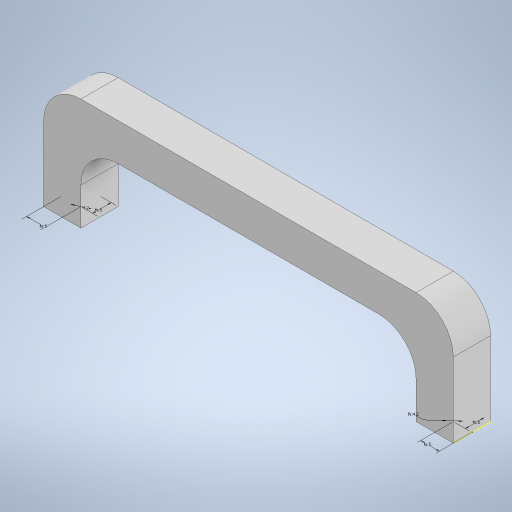
# Autodesk Inventor part: side door handle v02
Saved by Autodesk Inventor 2023 (Build 270158000, 158)
## iProperties
Created: 2024-06-24
Part Number: side door handle v02
Material: Generic
Document SubType Name: Modeling
Designer: Akramilab
Density: 1 g/cm^3
Appearance: Default
Author: Akramilab
Autodesk Inventor part; units mm, degrees
ref_plane "YZ Plane" through (0, 0, 0) normal (1, 0, 0) x (0, 1, 0)
ref_plane "XZ Plane" through (0, 0, 0) normal (0, 1, 0) x (-1, 0, 0)
ref_plane "XY Plane" through (0, 0, 0) normal (0, 0, 1) x (1, 0, 0)
sketch "Sketch1" plane through (0, 0, 0) normal (0, 0, 1) x (1, 0, 0)
  line L0 (0, 0) -> (110, 0)
  line L1 (110, 0) -> (110, -30)
  line L2 (110, -30) -> (0, -30)
  line L3 (0, -30) -> (0, 0)
  line L4 (10, -30) -> (100, -30)
  line L5 (100, -30) -> (100, -10)
  line L6 (100, -10) -> (10, -10)
  line L7 (10, -10) -> (10, -30)
  point P0 (0, -15)
  point P1 (55, 0)
  dimension "d0" = 110
  dimension "d1" = 30
  dimension "d2" = 10
  dimension "d3" = 10
  dimension "d4" = 10
  constraints: 16 end point, 4 parallel, 2 horizontal, 2 midpoint, 2 perpendicular, 1 point on line
  measures "d0" distance of L1.end L2.end
  measures "d1" distance of L0.end L1.end
  measures "d2" distance from line of L7 point (0, -15)
  measures "d3" distance between parallel lines of L1 L5
  measures "d4" distance from line of L6 point (55, 0)
extrude "Extrusion1" add sketch "Sketch1" along normal blind 10 contours L0 L1 L2 L5 L6 L7 L3
fillet "Fillet1" radius 10 4 edges at (0, 0, 5) (110, 0, 5) (10, -10, 5) (100, -10, 5)
sketch "Sketch2" plane through (0, -30, 0) normal (0, -1, 0) x (1, 0, 0)
  line L0 (0, 0) -> (10, 0) projected
  line L1 (0, 0) -> (0, 10) projected
  circle A0 centre (5, 5) radius 2.1
  line L2 (110, 0) -> (110, 10) projected
  line L3 (100, 0) -> (110, 0) projected
  circle A1 centre (104.6302, 5) radius 2.1
  point P0 (5, 0)
  point P1 (0, 5)
  point P2 (105, 5)
  point P3 (110, 5)
  dimension "d8" = 5
  dimension "d9" = 5
  dimension "d10" = 4.2
  dimension "d11" = 5
  dimension "d12" = 5
  dimension "d13" = 4.2
  constraints: 3 midpoint, 2 centre point, 1 coincident
  measures "d8" distance of point (5, 0) point (5, 5)
  measures "d9" distance of point (5, 5) point (0, 5)
  measures "d10" diameter of A0
  measures "d11" distance of point (110, 5) point (105, 5)
  measures "d12" distance from line of L3 point (105, 5)
  measures "d13" diameter of A1
equation "\"d3\" = d2"
equation "\"d4\" = d2"
equation "\"d5\" = d2"
equation "\"d8\" = 0.5 * d2"
equation "\"d9\" = 0.5 * d2"
equation "\"d11\" = d9"
equation "\"d12\" = d8"
equation "\"d13\" = d10"
body "Solid1"
